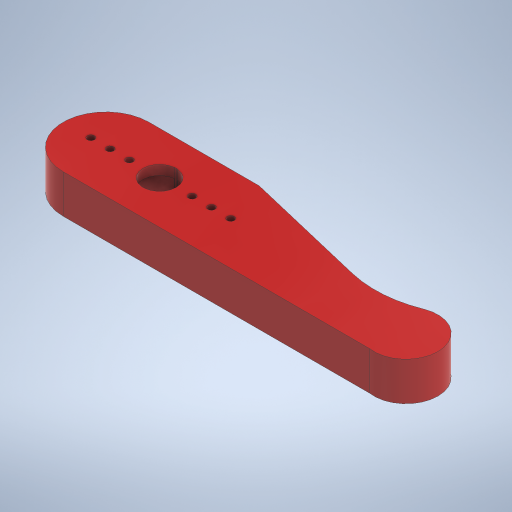
# Autodesk Inventor part: patanueva2
Saved by Autodesk Inventor 2024.3 (Build 283343000, 343)
## iProperties
Created: 2025-08-09
Part Number: patanueva2
Material: Generic
Document SubType Name: Modeling
Designer: jscme
Density: 1 g/cm^3
Appearance: Default
Author: jscme
Autodesk Inventor part; units mm, degrees
ref_plane "YZ Plane" through (0, 0, 0) normal (1, 0, 0) x (0, 1, 0)
ref_plane "XZ Plane" through (0, 0, 0) normal (0, 1, 0) x (-1, 0, 0)
ref_plane "XY Plane" through (0, 0, 0) normal (0, 0, 1) x (1, 0, 0)
sketch "Sketch1" plane through (0, 0, 0) normal (0, 1, 0) x (-1, 0, 0)
  line L0 (-3.0181, -8.89) -> (-25.8781, -8.89)
  line L1 (-3.0181, 8.89) -> (-27.578, 8.89)
  line L2 (-25.8781, -8.89) -> (-51.2781, -2.8161)
  line L3 (-27.578, 8.89) -> (-53.0779, 8.89)
  arc A0 (-51.2781, -2.8161) -> (-65.0775, -3.8214) centre (-56.5948, -25.0493) ccw
  line L4 (-53.0779, 8.89) -> (-66.5181, 8.89)
  arc A1 (-66.5181, 8.89) -> (-65.0775, -3.8214) centre (-67.5384, 2.337) ccw
  arc A2 (-3.0181, -8.89) -> (-3.0181, 8.89) centre (-3.0181, 0) ccw
  point P0 (0, 0)
  point P1 (-74.1281, 1.5902)
  point P2 (5.8719, 0)
  dimension "d31" = 80
  dimension "d32" = 8.89
  dimension "d33" = 6.6319
  dimension "d35" = 25.4
  dimension "d36" = 63.5
  dimension "d37" = 22.86
  dimension "d38" = 22.86
  constraints: 10 end point, 8 point on circle, 4 horizontal, 4 tangent, 3 centre point, 1 horizontal alignment
  measures "d31" horizontal distance of point (-74.128, 1.59) point (5.872, 0)
  measures "d32" radius of A2
  measures "d33" radius of A1
  measures "d35" horizontal distance of L0.end L2.end
  measures "d36" distance of L4.end L1.start
  measures "d37" distance of L0.start L0.end
  measures "d38" radius of A0
extrude "Extrusion1" add sketch "Sketch1" along normal blind 8
sketch "Sketch3" plane through (0, 8, 0) normal (0, 1, 0) x (1, 0, 0)
  circle A0 centre (14.1281, 0) radius 3.429
  arc A1 (3.0181, 8.89) -> (3.0181, -8.89) centre (3.0181, 0) ccw projected
  line L0 (14.1281, 3.429) -> (-0.8719, 2.5603)
  line L1 (14.1281, -3.429) -> (-0.8805, -2.725)
  arc A2 (-0.8719, 2.5603) -> (-0.8805, -2.725) centre (-0.7188, -0.0826) ccw
  line L2 (14.1281, 5.8203) -> (14.1281, -4.2261)
  line L3 (14.1281, 3.429) -> (29.1281, 2.5603)
  line L4 (14.1281, -3.429) -> (29.1368, -2.725)
  arc A3 (29.1368, -2.725) -> (29.1281, 2.5603) centre (28.9751, -0.0826) ccw
  point P0 (-5.8719, 0)
  point P1 (-5.8719, 0)
  point P2 (14.1281, 0.7971)
  point P3 (25.2381, 0)
  point P4 (14.4491, -3.4139)
  point P5 (14.524, 3.4061)
  point P6 (13.7323, 3.4061)
  point P7 (13.8072, -3.4139)
  dimension "d40" = 20
  dimension "d41" = 15
  dimension "d42" = 15.0086
  dimension "d43" = 6
  dimension "d56" = 6.858
  constraints: 10 end point, 8 point on circle, 4 symmetric about line, 3 centre point, 3 vertical alignment, 1 equal length, 1 horizontal alignment, 1 midpoint, 1 tangent, 1 vertical, 1 other
  measures "d40" distance of point (-5.872, 0) A0.centre
  measures "d41" horizontal distance of L0.start L0.end
  measures "d42" horizontal distance of L1.start L1.end
  measures "d43" angle of L1 L0
  measures "d56" diameter of A0
extrude "Extrusion2" cut sketch "Sketch3" against normal through all contours L2 L3 A0 | A0 L0 L2
sketch "Sketch5" plane through (0, 0, 0) normal (0, -1, 0) x (1, 0, 0)
  circle A0 centre (14.1281, 0) radius 3.429
  line L0 (14.1281, 3.429) -> (-0.8719, 2.5603)
  line L1 (14.1281, -3.429) -> (-0.8805, -2.725)
  arc A1 (-0.8719, 2.5603) -> (-0.8805, -2.725) centre (-0.7188, -0.0826) ccw
  line L2 (14.1281, 5.8203) -> (14.1281, -4.2261)
  arc A2 (29.1368, -2.725) -> (29.1281, 2.5603) centre (28.9751, -0.0826) ccw
  line L3 (14.1281, 3.429) -> (29.1281, 2.5603)
  line L4 (14.1281, -3.429) -> (29.1368, -2.725)
  arc A3 (3.0181, 8.89) -> (3.0181, -8.89) centre (3.0181, 0) ccw projected
  point P0 (0, 0)
  point P1 (3.2251, 0.6634)
  point P2 (14.1281, 0.7971)
  point P3 (25.0312, 0.6634)
  point P4 (13.8072, -3.4139)
  point P5 (13.7323, 3.4061)
  point P6 (14.524, 3.4061)
  point P7 (14.4491, -3.4139)
  point P8 (-5.8719, 0)
  dimension "d58" = 15.0086
  dimension "d59" = 6
  dimension "d60" = 6.858
  dimension "d77" = 20
  constraints: 10 end point, 7 point on circle, 4 symmetric about line, 3 centre point, 3 vertical alignment, 1 coincident, 1 equal length, 1 horizontal alignment, 1 midpoint, 1 tangent, 1 vertical, 1 other
  measures "d58" horizontal distance of L1.start L1.end
  measures "d59" angle of L1 L0
  measures "d60" diameter of A0
  measures "d77" distance of point (-5.872, 0) A0.centre
extrude "Extrusion5" cut sketch "Sketch5" against normal blind 6 contours L1 A1 L0 A0 | A0 L3 A2 L4
sketch "Sketch6" plane through (0, 0, 0) normal (0, -1, 0) x (1, 0, 0)
  circle A0 centre (14.2886, 0) radius 3.429
  line L0 (14.2886, 3.429) -> (-0.7114, 2.5603)
  line L1 (14.2886, -3.429) -> (-0.72, -2.725)
  arc A1 (-0.7114, 2.5603) -> (-0.72, -2.725) centre (-0.5583, -0.0826) ccw
  line L2 (14.2886, 4.0046) -> (14.2886, -6.0418)
  arc A2 (29.2973, -2.725) -> (29.2886, 2.5603) centre (29.1356, -0.0826) ccw
  line L3 (14.2886, 3.429) -> (29.2886, 2.5603)
  line L4 (14.2886, -3.429) -> (29.2973, -2.725)
  circle A3 centre (7.7915, -0.0783) radius 0.75
  circle A4 centre (3.7915, -0.0783) radius 0.75
  circle A5 centre (-0.2085, -0.0783) radius 0.75
  circle A6 centre (20.7857, -0.0783) radius 0.75
  circle A7 centre (24.7857, -0.0783) radius 0.75
  circle A8 centre (28.7857, -0.0783) radius 0.75
  line L5 (14.1281, 3.429) -> (14.4491, 3.4139) projected
  point P0 (0, 0)
  point P1 (-3.6617, 0)
  point P2 (-5.7114, 0)
  point P3 (14.2886, -1.0186)
  point P4 (36.3588, -1.6825)
  point P5 (1.283, -0.0783)
  point P6 (-3.2057, -0.0783)
  point P7 (14.2886, 3.4215)
  dimension "d63" = 20
  dimension "d64" = 15
  dimension "d65" = 15.0086
  dimension "d66" = 6
  dimension "d67" = 6.858
  dimension "d68" = 6
  dimension "d69" = 1.5
  dimension "d70" = 1.5
  dimension "d71" = 1.5
  dimension "d72" = 4
  dimension "d73" = 4
  dimension "d74" = 2.9972
  constraints: 10 end point, 9 centre point, 7 point on circle, 7 symmetric about line, 6 horizontal alignment, 4 vertical alignment, 2 midpoint, 1 equal length, 1 tangent, 1 vertical, 4 other
  measures "d63" distance of point (-5.711, 0) A0.centre
  measures "d64" horizontal distance of L3.start L0.end
  measures "d65" horizontal distance of L4.start L1.end
  measures "d66" angle of L1 L0
  measures "d67" diameter of A0
  measures "d68" angle of L4 L3
  measures "d69" diameter of A5
  measures "d70" diameter of A4
  measures "d71" diameter of A3
  measures "d72" distance of A5.centre A4.centre
  measures "d73" distance of A4.centre A3.centre
  measures "d74" distance of point (-3.206, -0.078) A5.centre
extrude "Extrusion6" cut sketch "Sketch6" against normal blind 25.4 contours A3 | A4 | A5 | A6 | A7 | A8
body "Solid1"
